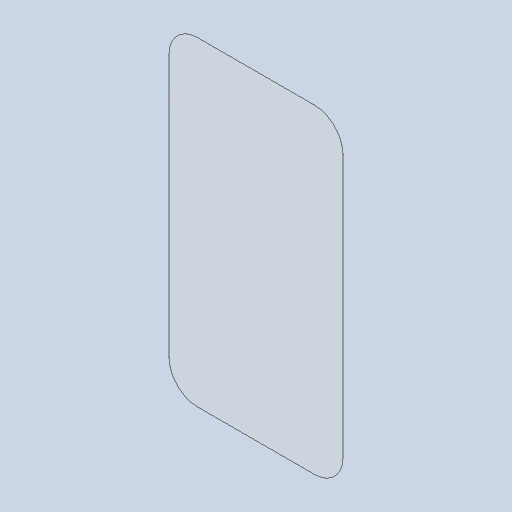
# Autodesk Inventor part: PLatico
Saved by Autodesk Inventor 2022.4 (Build 264492000, 492)
## iProperties
Created: 2022-11-28
Part Number: PLatico
Material: Plastic, Transparent
Document SubType Name: Modeling
Designer: David
Density: 1.188 g/cm^3
Appearance: Transparent - Clear
Author: David
Autodesk Inventor part; units mm, degrees
ref_plane "YZ Plane" through (0, 0, 0) normal (1, 0, 0) x (0, 1, 0)
ref_plane "XZ Plane" through (0, 0, 0) normal (0, 1, 0) x (-1, 0, 0)
ref_plane "XY Plane" through (0, 0, 0) normal (0, 0, 1) x (1, 0, 0)
sketch "Sketch1" plane through (0, 0, 0) normal (0, 0, 1) x (1, 0, 0)
  line L0 (-300, -1100) -> (900, -1100)
  line L1 (900, -1100) -> (900, 850)
  line L2 (900, 850) -> (-300, 850)
  line L3 (-300, 850) -> (-300, -1100)
  line L4 (-300, -1100) -> (900, 850) construction
  line L5 (900, -1100) -> (-300, 850) construction
  line L6 (0, 700) -> (600, 700)
  line L7 (750, 550) -> (750, -800)
  line L8 (600, -950) -> (0, -950)
  line L9 (-150, -800) -> (-150, 550)
  arc A0 (750, 550) -> (600, 700) centre (600, 550) ccw
  arc A1 (0, 700) -> (-150, 550) centre (0, 550) ccw
  arc A2 (-150, -800) -> (0, -950) centre (0, -800) ccw
  arc A3 (600, -950) -> (750, -800) centre (600, -800) ccw
  line L10 (600, 697) -> (0, 697)
  arc A4 (0, 697) -> (-147, 550) centre (0, 550) ccw
  line L11 (-147, 550) -> (-147, -800)
  arc A5 (-147, -800) -> (0, -947) centre (0, -800) ccw
  line L12 (0, -947) -> (600, -947)
  arc A6 (600, -947) -> (747, -800) centre (600, -800) ccw
  line L13 (747, -800) -> (747, 550)
  arc A7 (747, 550) -> (600, 697) centre (600, 550) ccw
  point P0 (0, 0)
  point P1 (0, 0)
  point P2 (300, -125)
  dimension "d0" = 1200
  dimension "d1" = 1950
  dimension "d2" = 150
  dimension "d3" = 150
  dimension "d4" = 150
  dimension "d5" = 150
  dimension "d6" = 150
  dimension "d7" = 3
  dimension "d10" = 1644
  constraints: 28 end point, 16 point on circle, 8 centre point, 8 tangent, 6 parallel, 3 perpendicular, 2 midpoint, 1 horizontal, 10 other
  measures "d0" distance of L2.end L1.end
  measures "d1" distance of L1.end L0.end
  measures "d2" distance between parallel lines of L2 L6
  measures "d3" radius of A0
  measures "d4" radius of A1
  measures "d5" radius of A2
  measures "d6" radius of A3
  measures "d7" distance between parallel lines of L6 L10
  measures "d10" distance between parallel lines of L12 L10
extrude "Extrusion1" add sketch "Sketch1" along normal mid plane 2 contours A7 L13 A6 L12 A5 L11 A4 L10
equation "\"Space7\" = 0"
body "Solid1"
